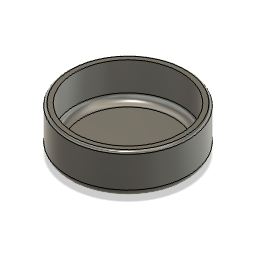
Revo GPS Lid (Autodesk Fusion 360 design; units mm, degrees)
Autodesk Fusion 360 part; units mm, degrees
sketch "Sketch1" plane through (0, 0, 0) normal (0, 1, 0) x (1, 0, 0)
  circle A0 centre (0, 0) radius 22.15
  circle A1 centre (0, 0) radius 25
  dimension "d1" = 44.3
  constraint coincident A0.centre A1.centre
  measures "d1" diameter of A0
extrude "Extrude1" add sketch "Sketch1" along normal blind 2 contours A0 | A1 makes body 1
extrude "Extrude2" add sketch "Sketch1" along normal blind 17 separate body makes body 2
fillet "Fillet3" radius 1 1 edges at (-23.3082, 17, 9.0404) on bodies 2
sketch "Sketch2" plane through (0, 0, 0) normal (0, 1, 0) x (1, 0, 0)
  line L0 (11.4048, -4.6211) -> (-11.4603, -4.6211) construction
  line L1 (-11.4603, -4.6211) -> (-11.4603, 16.7283) construction
  line L2 (-11.4603, 16.7283) -> (11.4048, 16.7283) construction
  line L3 (11.4048, 16.7283) -> (11.4048, -4.6211) construction
  dimension "d12" = 10
  text T0 "^\nGPS" font "Arial" height 10 align centre middle in box 22.8651 x 21.3494 at (11.4048, -4.6211) x (-1, 0) y (0, 1) spacing 1
extrude "Extrude3" add sketch "Sketch2" against normal blind 1.2 text T0 bodies 1
fillet "Fillet4" radius 1 7 edges at (-0.8531, 0, -15.6) (-2.3129, 0, -13.5638) (2.2574, 0, -13.5638) (0.8079, 0, -15.6) (1.6844, 0, -16.2958) (-1.7194, 0, -16.2958) (-0.0141, 0, -19.0277) on bodies 1
combine "Combine1" operation add target body 1 tool bodies 2
fillet "Fillet5" radius 3 1 edges at (-20.6511, 2, 8.0098) on bodies 1
fillet "Fillet6" radius 3 1 edges at (-23.3082, 0, 9.0404) on bodies 1
